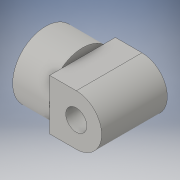
# Autodesk Inventor part: Germi01-03-01
Saved by Autodesk Inventor 2016 (Build 200138000, 138)
## iProperties
Created: 2016-11-08
Part Number: Germi01-03-01
Material: Generic
Document SubType Name: Modeling
Designer: Kai
Density: 1 g/cm^3
Appearance: Default
Author: Kai
Autodesk Inventor part; units mm, degrees
ref_plane "YZ Plane" through (0, 0, 0) normal (1, 0, 0) x (0, 1, 0)
ref_plane "XZ Plane" through (0, 0, 0) normal (0, 1, 0) x (-1, 0, 0)
ref_plane "XY Plane" through (0, 0, 0) normal (0, 0, 1) x (1, 0, 0)
sketch "Sketch1" plane through (0, 0, 0) normal (0, 1, 0) x (-1, 0, 0)
  line L0 (0, 15.4608) -> (12.8016, 15.4608)
  line L1 (12.8016, 15.4608) -> (12.8016, -0.338)
  line L2 (12.8016, -0.338) -> (0, -0.338)
  line L3 (0, -0.338) -> (0, 15.4608)
  constraints: 8 end point, 2 horizontal, 1 perpendicular, 1 vertical
extrude "Extrusion1" add sketch "Sketch1" along normal blind 12.192
sketch "Sketch2" plane through (-12.8016, 0, 15.4608) normal (0, 0, 1) x (1, 0, 0)
  arc A0 (6.4008, 0) -> (6.4008, 12.192) centre (6.4008, 6.096) ccw
  line L0 (0, 12.192) -> (12.8016, 12.192) projected
  line L1 (12.8016, 0) -> (0, 0) projected
  line L2 (6.4008, 0) -> (17.5033, -4.1356)
  line L3 (17.5033, -4.1356) -> (19.4121, 8.0167)
  line L4 (19.4121, 8.0167) -> (11.5072, 13.7088)
  line L5 (11.5072, 13.7088) -> (6.4008, 12.192)
  constraints: 8 end point, 2 midpoint, 2 point on circle, 1 centre point, 1 tangent
extrude "Extrusion2" cut sketch "Sketch2" along normal mid plane 2540
sketch "Sketch3" plane through (-12.8016, 0, 15.4608) normal (0, 0, 1) x (1, 0, 0)
  arc A0 (6.4008, 0) -> (6.4008, 12.192) centre (6.4008, 6.096) ccw projected
  circle A1 centre (6.4008, 6.096) radius 2.54
  point P0 (12.8016, 0)
  dimension "d8" = 5.08
  constraints: 1 centre point, 1 coincident
  measures "d8" diameter of A1
extrude "Extrusion3" cut sketch "Sketch3" against normal blind 2540
sketch "Sketch4" plane through (-12.8016, 0, -0.338) normal (-1, 0, 0) x (0, 0, 1)
  circle A0 centre (7.8994, 6.096) radius 7.8994
  point P0 (0.338, 0)
  constraints: 1 centre point
extrude "Extrusion4" add sketch "Sketch4" along normal blind 8.89
body "Solid1"
